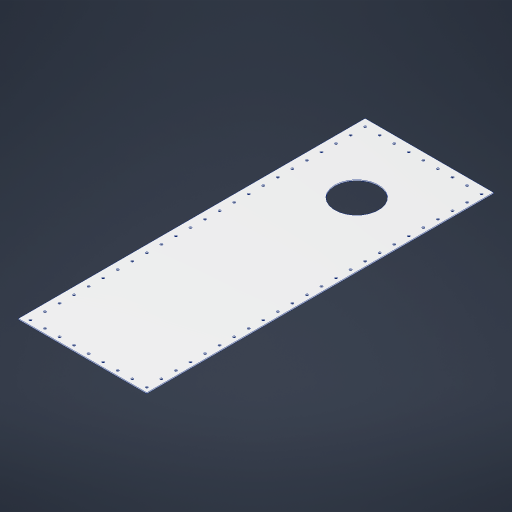
# Autodesk Inventor part: EBox-BottomPlate
Saved by Autodesk Inventor 2023 (Build 270158000, 158)
## iProperties
Created: 2023-01-19
Part Number: EBox-BottomPlate
Material: Aluminum 6061
Document SubType Name: Modeling
Designer: Nebil
Density: 2.7 g/cm^3
Appearance: Aluminum - Flat
Author: Nebil
Autodesk Inventor part; units mm, degrees
ref_plane "YZ Plane" through (0, 0, 0) normal (1, 0, 0) x (0, 1, 0)
ref_plane "XZ Plane" through (0, 0, 0) normal (0, 1, 0) x (-1, 0, 0)
ref_plane "XY Plane" through (0, 0, 0) normal (0, 0, 1) x (1, 0, 0)
sketch "Sketch1" plane through (0, 0, 0) normal (0, 1, 0) x (-1, 0, 0)
  line L0 (-112.014, 302.514) -> (112.014, 302.514)
  line L1 (112.014, 302.514) -> (112.014, -302.514)
  line L2 (112.014, -302.514) -> (-112.014, -302.514)
  line L3 (-112.014, -302.514) -> (-112.014, 302.514)
  line L4 (-112.014, 302.514) -> (112.014, -302.514) construction
  line L5 (112.014, 302.514) -> (-112.014, -302.514) construction
  circle A0 centre (99.314, -289.814) radius 2.0701
  circle A1 centre (73.914, -289.814) radius 2.0701
  circle A2 centre (48.514, -289.814) radius 2.0701
  circle A3 centre (23.114, -289.814) radius 2.0701
  circle A4 centre (-2.286, -289.814) radius 2.0701
  circle A5 centre (-27.686, -289.814) radius 2.0701
  circle A6 centre (-53.086, -289.814) radius 2.0701
  circle A7 centre (-78.486, -289.814) radius 2.0701
  circle A8 centre (-103.886, -289.814) radius 2.0701
  circle A9 centre (99.314, -264.414) radius 2.0701
  circle A10 centre (99.314, -239.014) radius 2.0701
  circle A11 centre (99.314, -213.614) radius 2.0701
  circle A12 centre (99.314, -188.214) radius 2.0701
  circle A13 centre (99.314, -162.814) radius 2.0701
  circle A14 centre (99.314, -137.414) radius 2.0701
  circle A15 centre (99.314, -112.014) radius 2.0701
  circle A16 centre (99.314, -86.614) radius 2.0701
  circle A17 centre (99.314, -61.214) radius 2.0701
  circle A18 centre (99.314, -35.814) radius 2.0701
  circle A19 centre (99.314, -10.414) radius 2.0701
  circle A20 centre (99.314, 14.986) radius 2.0701
  circle A21 centre (99.314, 40.386) radius 2.0701
  circle A22 centre (99.314, 65.786) radius 2.0701
  circle A23 centre (99.314, 91.186) radius 2.0701
  circle A24 centre (99.314, 116.586) radius 2.0701
  circle A25 centre (99.314, 141.986) radius 2.0701
  circle A26 centre (99.314, 167.386) radius 2.0701
  circle A27 centre (99.314, 192.786) radius 2.0701
  circle A28 centre (99.314, 218.186) radius 2.0701
  circle A29 centre (99.314, 243.586) radius 2.0701
  circle A30 centre (99.314, 268.986) radius 2.0701
  circle A31 centre (99.314, 294.386) radius 2.0701
  circle A32 centre (73.914, 294.386) radius 2.0701
  circle A33 centre (48.514, 294.386) radius 2.0701
  circle A34 centre (23.114, 294.386) radius 2.0701
  circle A35 centre (-2.286, 294.386) radius 2.0701
  circle A36 centre (-27.686, 294.386) radius 2.0701
  circle A37 centre (-53.086, 294.386) radius 2.0701
  circle A38 centre (-78.486, 294.386) radius 2.0701
  circle A39 centre (-103.886, 294.386) radius 2.0701
  circle A40 centre (-103.886, 268.986) radius 2.0701
  circle A41 centre (-103.886, 243.586) radius 2.0701
  circle A42 centre (-103.886, 218.186) radius 2.0701
  circle A43 centre (-103.886, 192.786) radius 2.0701
  circle A44 centre (-103.886, 167.386) radius 2.0701
  circle A45 centre (-103.886, 141.986) radius 2.0701
  circle A46 centre (-103.886, 116.586) radius 2.0701
  circle A47 centre (-103.886, 91.186) radius 2.0701
  circle A48 centre (-103.886, 65.786) radius 2.0701
  circle A49 centre (-103.886, 40.386) radius 2.0701
  circle A50 centre (-103.886, 14.986) radius 2.0701
  circle A51 centre (-103.886, -10.414) radius 2.0701
  circle A52 centre (-103.886, -35.814) radius 2.0701
  circle A53 centre (-103.886, -61.214) radius 2.0701
  circle A54 centre (-103.886, -86.614) radius 2.0701
  circle A55 centre (-103.886, -112.014) radius 2.0701
  circle A56 centre (-103.886, -137.414) radius 2.0701
  circle A57 centre (-103.886, -162.814) radius 2.0701
  circle A58 centre (-103.886, -188.214) radius 2.0701
  circle A59 centre (-103.886, -213.614) radius 2.0701
  circle A60 centre (-103.886, -239.014) radius 2.0701
  circle A61 centre (-103.886, -264.414) radius 2.0701
  circle A62 centre (-0.2159, -175.514) radius 38.1
  point P0 (0, 0)
  dimension "d0" = 605.028
  dimension "d1" = 224.028
  dimension "d5" = 4.1402
  dimension "d6" = 12.7
  dimension "d7" = 12.7
  dimension "d10" = 25.4
  dimension "d17" = 25.4
  dimension "d24" = 25.4
  dimension "d31" = 25.4
  dimension "d36" = 76.2
  dimension "d37" = 127
  constraints: 63 centre point, 12 end point, 3 horizontal, 2 midpoint, 2 parallel, 2 vertical, 1 perpendicular, 122 other
  measures "d0" distance of L0.end L1.end
  measures "d1" distance of L1.end L2.end
  measures "d5" diameter of A0
  measures "d6" distance from line of A0.centre L2
  measures "d7" distance from line of L1 A0.centre
  measures "d10" distance of A0.centre A1.centre
  measures "d17" distance of A0.centre A9.centre
  measures "d24" distance of A31.centre A32.centre
  measures "d31" distance of A39.centre A40.centre
  measures "d36" diameter of A62
  measures "d37" distance from line of A62.centre L2
extrude "Extrusion1" add sketch "Sketch1" along normal blind 1.5875
body "Solid1"
